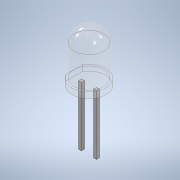
# Autodesk Inventor part: OPE5594A
Saved by Autodesk Inventor 2021 (Build 250183000, 183)
## iProperties
Created: 2021-06-29
Part Number: OPE5594A
Material: Generic
Document SubType Name: Modeling
Designer: ermoz
Density: 1 g/cm^3
Appearance: Default
Author: ermoz
Autodesk Inventor part; units mm, degrees
ref_plane "YZ Plane" through (0, 0, 0) normal (1, 0, 0) x (0, 1, 0)
ref_plane "XZ Plane" through (0, 0, 0) normal (0, 1, 0) x (-1, 0, 0)
ref_plane "XY Plane" through (0, 0, 0) normal (0, 0, 1) x (1, 0, 0)
sketch "Sketch1" plane through (0, 0, 0) normal (1, 0, 0) x (0, 1, 0)
  arc A0 (2.5, 0) -> (0, 2.5) centre (0, 0) ccw
  line L0 (-5.2, 0) -> (-5.2, 2.5)
  line L1 (-5.2, 2.5) -> (0, 2.5)
  line L2 (-5.2, 0) -> (2.5, 0)
  dimension "d0" = 2.5
  dimension "d1" = 7.7
  constraints: 6 end point, 2 point on circle, 1 centre point, 1 coincident, 1 horizontal, 1 perpendicular, 1 vertical
  measures "d0" radius of A0
  measures "d1" distance from line of L0 L2.end
revolve "Revolution1" add sketch "Sketch1" angle 360 about axis through (0, -5.2, 0) along (0, 1, 0)
sketch "Sketch2" plane through (0, -5.2, 0) normal (0, -1, 0) x (1, 0, 0)
  circle A0 centre (0, 0) radius 2.85
  dimension "d3" = 5.7
  constraints: 1 centre point, 1 coincident
  measures "d3" diameter of A0
extrude "Extrusion1" add sketch "Sketch2" along normal blind 1
sketch "Sketch3" plane through (0, -6.2, 0) normal (0, -1, 0) x (1, 0, 0)
  circle A0 centre (0, 0) radius 2.5 projected
  line L0 (-2.5, 1.3684) -> (-2.5, -1.3684)
  circle A1 centre (0, 0) radius 2.85 projected
  constraints: 2 end point, 2 point on circle, 1 tangent, 1 vertical
extrude "Extrusion2" cut sketch "Sketch3" against normal up to surface (1 mm away) contours L0 A1 picked at (-2.5741, -0.7373)
sketch "Sketch4" plane through (0, -6.2, 0) normal (0, -1, 0) x (1, 0, 0)
  line L0 (1.5, -0.25) -> (1, -0.25)
  line L1 (1, -0.25) -> (1, 0.25)
  line L2 (1, 0.25) -> (1.5, 0.25)
  line L3 (1.5, 0.25) -> (1.5, -0.25)
  line L4 (1.5, -0.25) -> (1, 0.25) construction
  line L5 (1, -0.25) -> (1.5, 0.25) construction
  line L6 (-1, -0.25) -> (-1.5, -0.25)
  line L7 (-1.5, -0.25) -> (-1.5, 0.25)
  line L8 (-1.5, 0.25) -> (-1, 0.25)
  line L9 (-1, 0.25) -> (-1, -0.25)
  line L10 (-1, -0.25) -> (-1.5, 0.25) construction
  line L11 (-1.5, -0.25) -> (-1, 0.25) construction
  line L12 (0, 0) -> (0, -1.2379)
  line L13 (0, 0) -> (-2.5, 0)
  point P0 (1.25, 0)
  point P1 (-1.25, 0)
  point P2 (-1.25, 0)
  point P3 (1.25, 0)
  point P4 (-1.25, 0)
  dimension "d8" = 2.5
  dimension "d9" = 0.5
  constraints: 28 end point, 8 midpoint, 5 perpendicular, 4 parallel, 3 horizontal, 1 horizontal alignment, 1 symmetric about line, 1 vertical
  measures "d8" distance of point (-1.25, 0) point (1.25, 0)
  measures "d9" distance of L2.end L0.start
extrude "Extrusion3" add sketch "Sketch4" along normal blind 10 separate body
body "Solid1"
body "Solid2"
